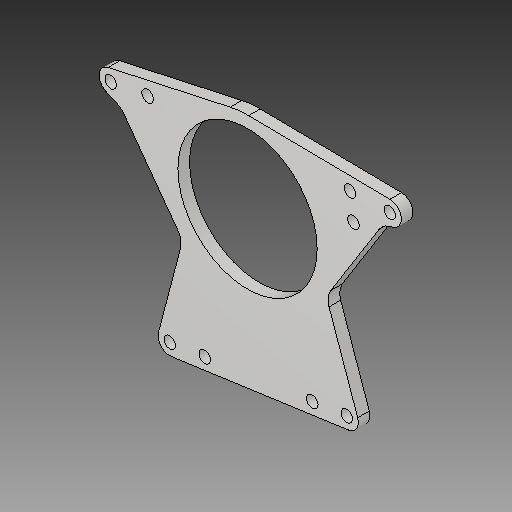
# Autodesk Inventor part: 中間フレーム内内
Saved by Autodesk Inventor 2019 (Build 230136000, 136)
## iProperties
Created: 2019-11-13
Part Number: 中間フレーム内内
Material: アルミニウム 2014-T4
Document SubType Name: Modeling
Designer: tanjihayato
Density: 2.8 g/cm^3
Appearance: サテン
Mass: 17.1133 g
Surface Area: 54.3894 cm^2
Volume: 6.11188 cm^3
Author: tanjihayato
Autodesk Inventor part; units mm, degrees
ref_plane "YZ Plane" through (0, 0, 0) normal (1, 0, 0) x (0, 1, 0)
ref_plane "XZ Plane" through (0, 0, 0) normal (0, 1, 0) x (-1, 0, 0)
ref_plane "XY Plane" through (0, 0, 0) normal (0, 0, 1) x (1, 0, 0)
sketch "スケッチ1" plane through (0, 0, 0) normal (0, 0, 1) x (1, 0, 0)
  circle A0 centre (0, 0) radius 20.55 construction
  circle A1 centre (-21.690847, -16.4118) radius 19.1 construction
  circle A2 centre (25.320198, -9.936175) radius 19.1 construction
  circle A3 centre (-50.601037, 30.814282) radius 1.5
  circle A4 centre (5.936242, 53.5882) radius 1.5
  circle A5 centre (27.390781, 10.682087) radius 1.5
  circle A6 centre (-42.891368, 18.388671) radius 1.5
  circle A7 centre (-21.690847, -16.4118) radius 4.025
  circle A8 centre (25.320198, -9.936175) radius 4.025
  circle A9 centre (0, 0) radius 4
  line L0 (-17.878475, -18.802579) -> (-30.416782, -38.796349) construction
  arc A10 (-17.878475, -18.802579) -> (-19.249319, -12.631728) centre (-21.690847, -16.4118) ccw construction
  line L1 (-19.249319, -12.631728) -> (-39.073694, 0.17273) construction
  line L2 (37.140856, -30.852246) -> (21.88658, -12.844829) construction
  arc A11 (22.365904, -6.541746) -> (21.88658, -12.844829) centre (25.320198, -9.936175) ccw construction
  line L3 (22.365904, -6.541746) -> (40.167798, 8.951885) construction
  line L4 (-21.690847, -16.4118) -> (-99.974162, 13.5882) construction
  line L5 (-105.525669, -16.4118) -> (-21.690847, -16.4118) construction
  line L6 (-21.690847, -16.4118) -> (-101.711328, -41.4118) construction
  line L7 (25.320198, -9.936175) -> (102.538646, -46.4118) construction
  line L8 (110.474331, -16.4118) -> (25.320198, -9.936175) construction
  line L9 (25.320198, -9.936175) -> (108.686903, 8.5882) construction
  line L10 (-18.05831, -13.755735) -> (-31.987893, 5.294901) construction
  line L11 (-17.338988, -17.556932) -> (-24.536725, -44.910558) construction
  line L12 (21.507701, -7.545597) -> (34.044954, 12.448834) construction
  line L13 (21.073936, -11.425892) -> (31.605914, -41.446035) construction
  arc A12 (-24.617584, -40.320148) -> (-19.506478, -44.416573) centre (-20.131998, -39.96026) ccw
  circle A13 centre (-20.131998, -39.96026) radius 3 construction
  arc A14 (-38.987898, 7.990671) -> (-39.33593, 8.526197) centre (-35.398239, 10.704405) ccw construction
  circle A15 centre (-35.398239, 10.704405) radius 3 construction
  arc A16 (-31.987893, 5.294901) -> (-33.846468, 6.774421) centre (-35.620429, 2.638836) ccw construction
  circle A17 centre (-41.515222, -3.607342) radius 1.5
  line L14 (-33.846468, 6.774421) -> (-56.065957, 16.305484) construction
  line L15 (-41.338636, 0.889192) -> (-72.631748, 2.118122) construction
  circle A18 centre (-42.891368, 18.388671) radius 3 construction
  circle A19 centre (-35.398239, 10.704405) radius 1.5
  circle A20 centre (36.773621, 17.534376) radius 1.5
  arc A21 (40.794171, 15.513193) -> (40.193362, 20.459332) centre (36.773621, 17.534376) ccw
  circle A22 centre (25.650815, -33.533859) radius 1.5
  arc A23 (26.276335, -37.990172) -> (30.150786, -33.517807) centre (25.650815, -33.533859) ccw
  circle A24 centre (36.773621, 17.534376) radius 3 construction
  circle A25 centre (25.650815, -33.533859) radius 3 construction
  arc A26 (36.683586, 14.402452) -> (34.044954, 12.448834) centre (37.857452, 10.058256) ccw construction
  line L16 (36.683586, 14.402452) -> (64.196789, 21.836927) construction
  line L17 (43.259945, 10.055344) -> (82.927317, 8.839597) construction
  circle A27 centre (27.390781, 10.682087) radius 3 construction
  circle A28 centre (-21.690847, -16.4118) radius 7.025 construction
  circle A29 centre (25.320198, -9.936175) radius 7.025 construction
  arc A30 (40.859312, 15.648342) -> (30.150786, -33.517807) centre (146.468505, -33.102887) ccw
  arc A31 (-24.617584, -40.320148) -> (-39.182737, 8.248399) centre (-145.115849, -49.987967) ccw
  arc A32 (-52.28241, 34.988367) -> (-54.190695, 28.100548) centre (-50.601037, 30.814282) ccw
  arc A33 (9.355983, 56.513156) -> (4.254869, 57.762285) centre (5.936242, 53.5882) ccw
  line L18 (-39.182737, 8.248399) -> (-54.190695, 28.100548)
  line L19 (-52.28241, 34.988367) -> (4.254869, 57.762285)
  line L20 (9.355983, 56.513156) -> (40.193362, 20.459332)
  line L21 (-19.506478, -44.416573) -> (26.276335, -37.990172)
  circle A34 centre (-20.131998, -39.96026) radius 1.5
  line L22 (-23.886768, -42.440522) -> (-17.338988, -17.556932)
  arc A35 (-17.338988, -17.556932) -> (-18.05831, -13.755735) centre (-21.690847, -16.4118) ccw
  line L23 (-18.05831, -13.755735) -> (-31.987893, 5.294901)
  arc A36 (-31.987893, 5.294901) -> (-33.846468, 6.774421) centre (-35.620429, 2.638836) ccw
  line L24 (-33.846468, 6.774421) -> (-40.094568, 9.454547)
  line L25 (40.797436, 15.514075) -> (36.683586, 14.402452)
  arc A37 (36.683586, 14.402452) -> (34.044954, 12.448834) centre (37.857452, 10.058256) ccw
  line L26 (34.044954, 12.448834) -> (21.507701, -7.545597)
  arc A38 (21.507701, -7.545597) -> (21.073936, -11.425892) centre (25.320198, -9.936175) ccw
  line L27 (21.073936, -11.425892) -> (29.592026, -35.70569)
  circle A39 centre (0, 0) radius 10.1 construction
  circle A40 centre (25.320198, -9.936175) radius 17.1 construction
  circle A41 centre (110.474331, -16.4118) radius 28.1 construction
  circle A42 centre (62.413099, -12.756939) radius 20.1 construction
  circle A43 centre (-21.690847, -16.4118) radius 17.1 construction
  circle A44 centre (-105.525669, -16.4118) radius 28.1 construction
  line L28 (-170.91498, -81.4118) -> (490.004419, -81.4118)
  line L29 (-105.525669, -16.4118) -> (-21.690847, -16.4118) construction
  line L30 (110.474331, -16.4118) -> (25.320198, -9.936175) construction
  line L31 (110.474331, -16.4118) -> (104.150058, -0.631953)
  line L32 (104.150058, -0.631953) -> (95.593688, 20.717252) construction
  line L33 (95.593688, 20.717252) -> (70.474331, -10.4118) construction
  line L34 (70.474331, -10.4118) -> (110.474331, -16.4118) construction
  line L35 (-137.681852, 53.5882) -> (165.818568, 53.5882)
  line L36 (25.320198, -9.936175) -> (108.686903, 8.5882) construction
  line L37 (25.320198, -9.936175) -> (102.538646, -46.4118) construction
  line L38 (25.320198, -9.936175) -> (5.936242, 53.5882) construction
  line L39 (5.936242, 53.5882) -> (127.64315, 30.26217)
  line L40 (127.64315, 30.26217) -> (110.474331, -16.4118) construction
  line L41 (102.538646, -46.4118) -> (118.068109, 0.832921) construction
  line L42 (118.068109, 0.832921) -> (5.936242, 53.5882) construction
  line L43 (108.686903, 8.5882) -> (129.858294, 53.5882) construction
  line L44 (129.858294, 53.5882) -> (5.936242, 53.5882) construction
  line L45 (119.272599, 31.0882) -> (366.444098, 68.5882) construction
  line L46 (119.05874, 6.925185) -> (362.021337, 65.824902) construction
  line L47 (110.303378, -22.78944) -> (351.062397, 44.553669) construction
  line L48 (127.64315, 30.26217) -> (4.192658, 19.461651) construction
  circle A45 centre (80.474331, 23.123973) radius 3 construction
  circle A46 centre (80.474331, 23.123973) radius 1.5
  arc A47 (79.800999, 27.573313) -> (76.161969, 24.409872) centre (80.474331, 23.123973) ccw
  circle A48 centre (70.474331, -10.4118) radius 1.5
  arc A49 (66.161969, -9.125901) -> (69.424217, -14.787558) centre (70.474331, -10.4118) ccw
  circle A50 centre (150.474331, 0.5882) radius 1.5
  arc A51 (152.562257, -3.398097) -> (154.040845, 3.33228) centre (150.474331, 0.5882) ccw
  circle A52 centre (127.64315, 30.26217) radius 1.5
  arc A53 (131.281576, 32.91016) -> (126.969818, 34.71151) centre (127.64315, 30.26217) ccw
  circle A54 centre (110.474331, -16.4118) radius 5
  arc A55 (108.607462, -24.190926) -> (114.186199, -23.49855) centre (110.474331, -16.4118) ccw
  line L49 (76.161969, 24.409872) -> (66.161969, -9.125901)
  line L50 (69.424217, -14.787558) -> (108.607462, -24.190926)
  line L51 (114.186199, -23.49855) -> (152.562257, -3.398097)
  line L52 (154.040845, 3.33228) -> (131.209664, 33.00625)
  line L53 (126.969818, 34.71151) -> (79.800999, 27.573313)
  circle A56 centre (-145.525669, 0.5882) radius 1.5
  arc A57 (-149.092184, 3.33228) -> (-147.613596, -3.398097) centre (-145.525669, 0.5882) ccw
  circle A58 centre (-105.525669, -16.4118) radius 5
  arc A59 (-109.237538, -23.49855) -> (-103.6588, -24.190926) centre (-105.525669, -16.4118) ccw
  circle A60 centre (-65.525669, -10.4118) radius 1.5
  arc A61 (-64.475556, -14.787558) -> (-61.213308, -9.125901) centre (-65.525669, -10.4118) ccw
  circle A62 centre (0, 0) radius 20.05 construction
  circle A63 centre (110.474331, -16.4118) radius 30.1 construction
  circle A64 centre (62.413099, -12.756939) radius 22.1 construction
  circle A65 centre (25.320198, -9.936175) radius 19.1 construction
  circle A66 centre (0, 0) radius 12.1 construction
  circle A67 centre (-21.690847, -16.4118) radius 19.1 construction
  circle A68 centre (-105.525669, -16.4118) radius 30.1 construction
  circle A69 centre (0, 0) radius 20.55 construction
  circle A70 centre (95.593688, 20.717252) radius 4.025 construction
  circle A71 centre (95.593688, 20.717252) radius 6.025 construction
  circle A72 centre (-75.525669, 23.123973) radius 1.5
  arc A73 (-71.213308, 24.409872) -> (-74.852338, 27.573313) centre (-75.525669, 23.123973) ccw
  circle A74 centre (-122.694488, 30.26217) radius 1.5
  arc A75 (-122.021157, 34.71151) -> (-126.261003, 33.00625) centre (-122.694488, 30.26217) ccw
  line L54 (-126.261003, 33.00625) -> (-149.092184, 3.33228)
  line L55 (-147.613596, -3.398097) -> (-109.237538, -23.49855)
  line L56 (-103.6588, -24.190926) -> (-64.475556, -14.787558)
  line L57 (-61.213308, -9.125901) -> (-71.213308, 24.409872)
  line L58 (-74.852338, 27.573313) -> (-122.021157, 34.71151)
  circle A76 centre (14, -17.4118) radius 2.29213 construction
  circle A77 centre (-14, -17.4118) radius 2.29213 construction
  circle A78 centre (-14, -17.4118) radius 14 construction
  circle A79 centre (14, -17.4118) radius 14 construction
  line L59 (-170.651239, -31.4118) -> (202.86558, -31.4118)
  line L60 (5.936242, 53.5882) -> (-42.252867, 34.177029) construction
  line L61 (5.936242, 53.5882) -> (-29.404465, 15.509095) construction
  circle A80 centre (5.936242, 53.5882) radius 1.5
  arc A81 (9.961109, 55.600773) -> (4.254869, 57.762285) centre (5.936242, 53.5882) ccw
  line L62 (-21.690847, -16.4118) -> (-99.974162, 13.5882) construction
  line L63 (-21.690847, -16.4118) -> (-101.711328, -41.4118) construction
  line L64 (9.961109, 55.600773) -> (31.415648, 12.694659)
  circle A82 centre (-50.601037, 30.814282) radius 1.5
  arc A83 (-52.28241, 34.988367) -> (-54.424801, 28.441767) centre (-50.601037, 30.814282) ccw
  line L65 (4.254869, 57.762285) -> (-52.28241, 34.988367)
  line L66 (-54.424801, 28.441767) -> (-46.715132, 16.016156)
  circle A84 centre (27.390781, 10.682087) radius 3 construction
  circle A85 centre (-84.86606, 5.271327) radius 4.5 construction
  circle A86 centre (-132.017427, -1.981251) radius 4.5 construction
  line L67 (-132.701548, 2.466443) -> (-85.550181, 9.71902) construction
  arc A87 (26.900287, 6.208898) -> (31.415648, 12.694659) centre (27.390781, 10.682087) ccw
  arc A88 (-46.715132, 16.016156) -> (-43.381863, 13.915483) centre (-42.891368, 18.388671) ccw
  line L68 (-43.381863, 13.915483) -> (26.900287, 6.208898)
  circle A89 centre (-42.252867, 34.177029) radius 3 construction
  circle A90 centre (25.320198, -9.936175) radius 4.025 construction
  circle A91 centre (-21.690847, -16.4118) radius 4.025 construction
  circle A92 centre (-42.891368, 18.388671) radius 1.5
  circle A93 centre (27.390781, 10.682087) radius 1.5
  circle A94 centre (-57.813011, 39.770535) radius 4.5 construction
  circle A95 centre (-99.303951, 63.315241) radius 4.5 construction
  line L69 (5.936242, 53.5882) -> (-35.940425, 22.842004) construction
  circle A96 centre (-58.005574, -24.479052) radius 20.1 construction
  circle A97 centre (-58.005574, -24.479052) radius 22.1 construction
  line L70 (-53.326057, 39.428119) -> (-56.279689, 0.724331) construction
  circle A98 centre (-42.252867, 34.177029) radius 4.5
  dimension "d127" = 9
  dimension "d128" = 9
  dimension "d143" = 9
  dimension "d0" = 8.05
  dimension "d1" = 8.05
  dimension "d2" = 8
  dimension "d3" = 20.968
  dimension "d4" = 20.968
  dimension "d5" = 17.3498
  dimension "d6" = 17.3498
  dimension "d7" = 16.8765
  dimension "d8" = 16.8765
  dimension "d9" = 20.9359
  dimension "d10" = 20.9359
  dimension "d11" = 9
  dimension "d12" = 6
  dimension "d13" = 9
  dimension "d14" = 6
  dimension "d15" = 9
  dimension "d16" = 20.968
  dimension "d17" = 20.968
  dimension "d18" = 6
  dimension "d19" = 3
  dimension "d20" = 3
  dimension "d21" = 9
  dimension "d22" = 3
  dimension "d23" = 9
  dimension "d24" = 6
  dimension "d25" = 6
  dimension "d26" = 9
  dimension "d27" = 16.8765
  dimension "d28" = 3
  dimension "d29" = 3
  dimension "d30" = 9
  dimension "d31" = 9
  dimension "d32" = 3
  dimension "d39" = 20.2
  dimension "d40" = 34.2
  dimension "d41" = 56.2
  dimension "d42" = 40.2
  dimension "d43" = 216
  dimension "d44" = 65
  dimension "d45" = 65
  dimension "d46" = 34.2
  dimension "d47" = 56.2
  dimension "d48" = 17
  dimension "d49" = 23
  dimension "d50" = 40
  dimension "d51" = 40
  dimension "d52" = 6
  dimension "d53" = 135
  dimension "d54" = 25
  dimension "d55" = 30
  dimension "d56" = 5
  dimension "d57" = 2
  dimension "d58" = 250
  dimension "d59" = 150
  dimension "d60" = 250
  dimension "d61" = 250
  dimension "d62" = 123.823
  dimension "d63" = 123.823
  dimension "d64" = 123.823
  dimension "d65" = 6
  dimension "d66" = 3
  dimension "d67" = 9
  dimension "d68" = 3
  dimension "d69" = 9
  constraints: 142 end point, 96 centre point, 70 tangent, 69 point on circle, 43 coincident, 13 equal length, 9 point on line, 5 horizontal, 3 midpoint, 2 collinear, 2 equal radius, 1 concentric, 1 parallel, 1 perpendicular, 13 other
  measures "d0" diameter of A7
  measures "d1" diameter of A8
  measures "d2" diameter of A9
  measures "d3" angle of L5 L4
  measures "d4" angle of L1 L10
  measures "d5" angle of L5 L6
  measures "d6" angle of L0 L11
  measures "d7" angle of L8 L9
  measures "d8" angle of L12 L3
  measures "d9" angle of L8 L7
  measures "d10" angle of L13 L2
  measures "d11" diameter of A12
  measures "d12" diameter of A13
  measures "d13" diameter of A14
  measures "d14" diameter of A15
  measures "d15" diameter of A16
  measures "d17" angle of L15 L14
  measures "d18" diameter of A18
  measures "d19" diameter of A19
  measures "d20" diameter of A20
  measures "d21" diameter of A21
  measures "d22" diameter of A22
  measures "d23" diameter of A23
  measures "d24" diameter of A24
  measures "d25" diameter of A25
  measures "d26" diameter of A26
  measures "d27" angle of L16 L17
  measures "d28" radial gap between concentric circles of A7 A28
  measures "d29" radial gap between concentric circles of A8 A29
  measures "d30" diameter of A32
  measures "d31" diameter of A33
  measures "d32" diameter of A34
  measures "d39" diameter of A39
  measures "d40" diameter of A40
  measures "d41" diameter of A41
  measures "d42" diameter of A42
  measures "d43" distance of L29.start L30.start
  measures "d44" distance from line of L28 L30.start
  measures "d45" distance from line of L28 L29.start
  measures "d46" diameter of A43
  measures "d47" diameter of A44
  measures "d48" distance of L30.start L31.end
  measures "d49" distance of L31.end L32.end
  measures "d50" distance of L32.end L33.end
  measures "d51" horizontal distance of L33.end L30.start
  measures "d52" vertical distance of L33.end L30.start
  measures "d53" distance between parallel lines of L28 L35
  measures "d54" vertical distance of L30.start L36.end
  measures "d55" vertical distance of L37.end L30.start
  measures "d56" angle of L40 L43
  measures "d57" angle of L40 L41
  measures "d58" distance of L45.start L45.end
  measures "d59" distance from line of L28 L45.end
  measures "d60" distance of L46.start L46.end
  measures "d61" distance of L47.start L47.end
  measures "d62" angle of L43 L45
  measures "d63" angle of L40 L46
  measures "d64" angle of L41 L47
  measures "d65" diameter of A45
  measures "d66" diameter of A46
  measures "d67" diameter of A47
  measures "d68" diameter of A48
  measures "d69" diameter of A49
sketch "スケッチ3" plane through (0, 0, 0) normal (0, 0, 1) x (1, 0, 0)
  line L0 (0, 0) -> (0, -41.46026)
  circle A0 centre (25.320198, -9.936175) radius 4.025
  circle A1 centre (25.650815, -33.533859) radius 1.5
  circle A2 centre (36.773621, 17.534376) radius 1.5
  arc A3 (41.059013, 16.161272) -> (32.782059, 19.61222) centre (36.773621, 17.534376) ccw
  line L1 (32.243549, -11.351383) -> (41.059013, 16.161272)
  line L2 (30.131291, -33.952594) -> (32.243549, -11.351383)
  arc A4 (21.183829, -34.077953) -> (30.131291, -33.952594) centre (25.650815, -33.533859) ccw
  line L3 (18.346737, -10.785566) -> (21.183829, -34.077953)
  arc A5 (19.088928, -6.692428) -> (18.346737, -10.785566) centre (25.320198, -9.936175) ccw
  line L4 (32.782059, 19.61222) -> (19.088928, -6.692428)
  circle A6 centre (-21.690847, -16.4118) radius 4.025
  circle A7 centre (-35.398239, 10.704405) radius 1.5
  circle A8 centre (-20.131998, -39.96026) radius 1.5
  arc A9 (-24.564595, -40.736203) -> (-15.635797, -40.145139) centre (-20.131998, -39.96026) ccw
  line L5 (-28.482017, -18.357797) -> (-24.564595, -40.736203)
  line L6 (-39.569097, 9.015043) -> (-28.482017, -18.357797)
  arc A10 (-31.564802, 13.061259) -> (-39.569097, 9.015043) centre (-35.398239, 10.704405) ccw
  line L7 (-15.706425, -12.732489) -> (-31.564802, 13.061259)
  arc A11 (-14.671778, -16.700416) -> (-15.706425, -12.732489) centre (-21.690847, -16.4118) ccw
  line L8 (-15.635797, -40.145139) -> (-14.671778, -16.700416)
  circle A12 centre (25.320198, -9.936175) radius 6
  circle A13 centre (-21.690847, -16.4118) radius 6
  constraints: 18 end point, 14 centre point, 12 point on circle, 2 coincident, 1 vertical
sketch "スケッチ2" plane through (0, 0, 0) normal (0, 0, 1) x (1, 0, 0)
  circle A0 centre (0, 0) radius 18
  circle A1 centre (-35.398239, 10.704405) radius 1.5
  line L0 (-33.846468, 6.774421) -> (-39.663363, 9.269581)
  arc A2 (-31.987893, 5.294901) -> (-33.846468, 6.774421) centre (-35.620429, 2.638836) ccw
  line L1 (-18.05831, -13.755735) -> (-31.987893, 5.294901)
  arc A3 (-17.338988, -17.556932) -> (-18.05831, -13.755735) centre (-21.690847, -16.4118) ccw
  line L2 (-17.338988, -17.556932) -> (-23.886768, -42.440522)
  line L3 (21.073936, -11.425892) -> (29.592026, -35.70569)
  arc A4 (21.507701, -7.545597) -> (21.073936, -11.425892) centre (25.320198, -9.936175) ccw
  line L4 (34.044954, 12.448834) -> (21.507701, -7.545597)
  arc A5 (36.683586, 14.402452) -> (34.044954, 12.448834) centre (37.857452, 10.058256) ccw
  line L5 (40.797436, 15.514075) -> (36.683586, 14.402452)
  circle A6 centre (36.773621, 17.534376) radius 1.5
  circle A7 centre (25.650815, -33.533859) radius 1.5
  circle A8 centre (-20.131998, -39.96026) radius 1.5
  arc A9 (-23.886768, -42.440522) -> (-19.506478, -44.416573) centre (-20.131998, -39.96026) ccw
  line L6 (-19.506478, -44.416573) -> (26.276335, -37.990172)
  arc A10 (26.276335, -37.990172) -> (29.592026, -35.70569) centre (25.650815, -33.533859) ccw
  circle A11 centre (27.390781, 10.682087) radius 1.5
  arc A12 (-36.154351, 15.140427) -> (-39.663363, 9.269581) centre (-35.398239, 10.704405) ccw
  arc A13 (40.794171, 15.513193) -> (36.647882, 22.032619) centre (36.773621, 17.534376) ccw
  arc A14 (-0.586782, 20.9918) -> (-3.528521, 20.701438) centre (0, 0) ccw
  line L7 (-36.154351, 15.140427) -> (-3.528521, 20.701438)
  line L8 (-0.586782, 20.9918) -> (36.647882, 22.032619)
  circle A15 centre (14, -17.4118) radius 14 construction
  circle A16 centre (-14, -17.4118) radius 14 construction
  line L9 (-170.651239, -31.4118) -> (202.86558, -31.4118)
  circle A17 centre (-11.072102, -38.688549) radius 3
  circle A18 centre (16.736705, -34.785107) radius 3
  circle A19 centre (26.477393, 17.246566) radius 3
  circle A20 centre (-25.835433, 12.334367) radius 3
  circle A21 centre (0, 0) radius 20.55 construction
  circle A22 centre (-25.835433, 12.334367) radius 1.5
  circle A23 centre (26.477393, 17.246566) radius 1.5
  circle A24 centre (16.736705, -34.785107) radius 1.5
  circle A25 centre (-11.072102, -38.688549) radius 1.5
  circle A26 centre (-11.072102, -38.688549) radius 4.5
  circle A27 centre (16.736705, -34.785107) radius 4.5
  circle A28 centre (26.477393, 17.246566) radius 4.5
  circle A29 centre (-25.835433, 12.334367) radius 4.5
  line L10 (32.782059, 19.61222) -> (19.088928, -6.692428)
  line L11 (-15.706425, -12.732489) -> (-31.564802, 13.061259)
  line L12 (-15.635797, -40.145139) -> (-14.671778, -16.700416)
  line L13 (18.346737, -10.785566) -> (21.183829, -34.077953)
  circle A30 centre (0, 0) radius 4
  dimension "d33" = 36
  dimension "d34" = 9
  dimension "d35" = 9
  dimension "d36" = 3
  dimension "d159" = 6
  dimension "d160" = 6
  dimension "d161" = 6
  dimension "d162" = 6
  dimension "d163" = 3
  dimension "d164" = 3
  dimension "d165" = 3
  dimension "d166" = 3
  dimension "d167" = 9
  dimension "d168" = 9
  dimension "d169" = 9
  dimension "d170" = 9
  dimension "d171" = 8
  constraints: 19 centre point, 12 coincident, 12 tangent, 10 point on circle, 8 end point, 2 point on line
  measures "d33" diameter of A0
  measures "d34" diameter of A12
  measures "d35" diameter of A13
  measures "d36" radial gap between concentric circles of A0 A14
  measures "d159" diameter of A17
  measures "d160" diameter of A18
  measures "d161" diameter of A19
  measures "d162" diameter of A20
  measures "d163" diameter of A22
  measures "d164" diameter of A23
  measures "d165" diameter of A24
  measures "d166" diameter of A25
  measures "d167" diameter of A26
  measures "d168" diameter of A27
  measures "d169" diameter of A28
  measures "d170" diameter of A29
  measures "d171" diameter of A30
extrude "押し出し1" add sketch "スケッチ2" along normal blind 3 contours A28 | A29 | L0 A12 L7 A14 L8 A13 L5 A5 L4 A4 L3 L9 A27 L2 A3 L1 A2 | L9 L12 A26 L6 A9 L2 | L9 A27 L6 A26 L12 | A27 L9 | L9 A27 | A26 | L9 L3 A10 L6 A27 | A17 | A18 | A19 | A20 | A22 | A23 | A24 | A25
extrude "押し出し2" cut sketch "スケッチ2" along normal blind 3 contours A22 | A23 | A24 | A25
sketch "スケッチ4" plane through (0, 0, 3) normal (0, 0, 1) x (1, 0, 0)
  circle A0 centre (26.477393, 17.246566) radius 1.5
  circle A1 centre (-11.072102, -38.688549) radius 1.5
  circle A2 centre (16.736705, -34.785107) radius 1.5
  circle A3 centre (-25.835433, 12.334367) radius 1.5
  circle A4 centre (0, 0) radius 18
  circle A5 centre (27.390781, 10.682087) radius 1.5
  circle A6 centre (-20.131998, -39.96026) radius 1.5
  circle A7 centre (25.650815, -33.533859) radius 1.5
  circle A8 centre (36.773621, 17.534376) radius 1.5
  circle A9 centre (-35.398239, 10.704405) radius 1.5
  line L0 (-39.663363, 9.269581) -> (-33.846468, 6.774421)
  arc A10 (-31.987893, 5.294901) -> (-33.846468, 6.774421) centre (-35.620429, 2.638836) ccw
  line L1 (-31.987893, 5.294901) -> (-18.05831, -13.755735)
  arc A11 (-17.338988, -17.556932) -> (-18.05831, -13.755735) centre (-21.690847, -16.4118) ccw
  line L2 (-17.338988, -17.556932) -> (-23.886768, -42.440522)
  arc A12 (-23.886768, -42.440522) -> (-19.506478, -44.416573) centre (-20.131998, -39.96026) ccw
  line L3 (-19.506478, -44.416573) -> (26.276335, -37.990172)
  arc A13 (26.276335, -37.990172) -> (29.592026, -35.70569) centre (25.650815, -33.533859) ccw
  line L4 (29.592026, -35.70569) -> (21.073936, -11.425892)
  arc A14 (21.507701, -7.545597) -> (21.073936, -11.425892) centre (25.320198, -9.936175) ccw
  line L5 (21.507701, -7.545597) -> (34.044954, 12.448834)
  arc A15 (36.683586, 14.402452) -> (34.044954, 12.448834) centre (37.857452, 10.058256) ccw
  line L6 (36.683586, 14.402452) -> (40.794171, 15.513193)
  arc A16 (40.794171, 15.513193) -> (36.647882, 22.032619) centre (36.773621, 17.534376) ccw
  line L7 (36.647882, 22.032619) -> (-0.586782, 20.9918)
  arc A17 (-0.586782, 20.9918) -> (-3.528521, 20.701438) centre (0, 0) ccw
  line L8 (-3.528521, 20.701438) -> (-36.154351, 15.140427)
  arc A18 (-36.154351, 15.140427) -> (-39.663363, 9.269581) centre (-35.398239, 10.704405) ccw
  arc A19 (-36.037367, 13.635534) -> (-36.58088, 7.947349) centre (-35.398239, 10.704405) ccw
  arc A20 (-23.033237, -39.196839) -> (-19.714985, -42.931136) centre (-20.131998, -39.96026) ccw
  arc A21 (26.067828, -36.504734) -> (28.481656, -32.540714) centre (25.650815, -33.533859) ccw
  arc A22 (37.556198, 14.638245) -> (36.811722, 20.534134) centre (36.773621, 17.534376) ccw
  line L9 (-19.714985, -42.931136) -> (26.067828, -36.504734)
  line L10 (36.647882, 22.032619) -> (-0.586782, 20.9918)
  arc A23 (0.266708, 20.998306) -> (-0.586782, 20.9918) centre (0, 0) ccw
  arc A24 (-3.528521, 20.701438) -> (-4.473897, 20.517901) centre (0, 0) ccw
  line L11 (-4.473897, 20.517901) -> (-36.037367, 13.635534)
  line L12 (0.266708, 20.998306) -> (36.811722, 20.534134)
  dimension "d174" = 6
  dimension "d175" = 6
  dimension "d176" = 6
  dimension "d177" = 6
  constraints: 12 point on circle, 6 centre point, 6 coincident, 6 end point, 6 tangent, 4 point on line
  measures "d174" diameter of A19
  measures "d175" diameter of A20
  measures "d176" diameter of A21
  measures "d177" diameter of A22
extrude "押し出し3" cut sketch "スケッチ4" against normal blind 10 contours A18 L8 A24 L11 A19 L0 | L7 A16 L6 A22 L12 A23 | A20 L9 A21 L4 A13 L3 A12 L2
equation "\"d4\" = d3"
equation "\"d6\" = d5"
equation "\"d8\" = d7"
equation "\"d10\" = d9"
equation "\"d16\" = d3"
equation "\"d17\" = d3"
equation "\"d27\" = d7"
equation "\"d46\" = d40"
equation "\"d47\" = d41"
equation "\"d63\" = d62"
equation "\"d64\" = d62"
